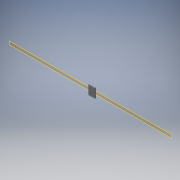
# Autodesk Inventor part: CarriagePlate
Saved by Autodesk Inventor 2019 (Build 230136000, 136)
## iProperties
Created: 2019-05-07
Part Number: CarriagePlate
Material: Generic
Document SubType Name: Modeling
Designer: Alex Jones
Density: 1 g/cm^3
Appearance: Default
Author: Alex Jones
Autodesk Inventor part; units mm, degrees
ref_plane "YZ Plane" through (0, 0, 0) normal (1, 0, 0) x (0, 1, 0)
ref_plane "XZ Plane" through (0, 0, 0) normal (0, 1, 0) x (-1, 0, 0)
ref_plane "XY Plane" through (0, 0, 0) normal (0, 0, 1) x (1, 0, 0)
ref_plane "Work Plane1" through (0, 0, 0) normal (0, 0, 1) x (1, 0, 0)
sketch "Sketch1" plane through (0, 0, 0) normal (0, 0, 1) x (1, 0, 0)
  circle A0 centre (-473.5705, 17.8) radius 2.5 projected
  circle A1 centre (-473.5705, 17.8) radius 9.9 construction
  circle A2 centre (-473.5705, -25) radius 2.5 projected
  circle A3 centre (-473.5705, -25) radius 9.9 construction
  line L0 (-473.5705, -25) -> (-473.5705, 17.8) construction
  circle A4 centre (-513.5705, 17.8) radius 2.5 projected
  circle A5 centre (-513.5705, 17.8) radius 9.9 construction
  circle A6 centre (-513.5705, -25) radius 2.5 projected
  circle A7 centre (-513.5705, -25) radius 9.9 construction
  line L1 (-513.5705, 17.8) -> (-513.5705, -25) construction
  line L2 (-513.5705, 17.8) -> (-473.5705, 17.8) construction
  line L3 (-513.5705, -25) -> (-473.5705, -25) construction
  line L4 (-463.5705, 27.8) -> (-463.5705, -35)
  line L5 (-463.5705, -35) -> (-523.5705, -35)
  line L6 (-523.5705, -35) -> (-523.5705, 27.8)
  line L7 (-523.5705, 27.8) -> (-463.5705, 27.8)
  point P0 (0, 0)
  dimension "d2" = 10
  constraints: 16 end point, 2 perpendicular, 1 horizontal, 1 vertical, 3 other
  measures "d2" distance between parallel lines of L2 L7
extrude "Extrusion1" add sketch "Sketch1" along normal blind 6.35
body "Solid1"
